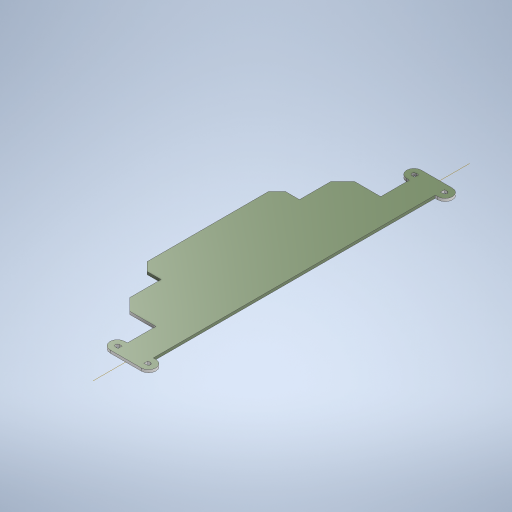
# Autodesk Inventor part: linefollower_chassy_model
Saved by Autodesk Inventor 2024 (Build 280153000, 153)
## iProperties
Created: 2024-02-06
Part Number: linefollower_chassy_model
Material: Generic
Document SubType Name: Modeling
Designer: kamil
Density: 1 g/cm^3
Appearance: Default
Author: kamil
Autodesk Inventor part; units mm, degrees
ref_plane "YZ Plane" through (0, 0, 0) normal (1, 0, 0) x (0, 1, 0)
ref_plane "XZ Plane" through (0, 0, 0) normal (0, 1, 0) x (-1, 0, 0)
ref_plane "XY Plane" through (0, 0, 0) normal (0, 0, 1) x (1, 0, 0)
sketch "Sketch1" plane through (0, 0, 0) normal (0, 1, 0) x (-1, 0, 0)
  line L0 (7.5, 90) -> (-7.5, 90)
  line L1 (-7.5, 90) -> (-7.5, -90)
  line L2 (-7.5, -90) -> (7.5, -90)
  line L3 (7.5, -90) -> (7.5, 90)
  line L4 (-7.5, 90) -> (7.5, -90) construction
  line L5 (-7.5, -90) -> (7.5, 90) construction
  line L6 (7.5, -90) -> (7.5, -81.5)
  line L7 (0, 90) -> (0, -90) construction
  line L8 (-7.5, 0) -> (7.5, 0) construction
  line L9 (7.5, -20.0447) -> (7.5, 20.0447)
  line L10 (7.5, 40) -> (37.5, 40)
  line L11 (42.5, 35) -> (42.5, -35)
  line L12 (37.5, -40) -> (7.5, -40)
  line L13 (7.5, -40) -> (7.5, 40)
  line L14 (-7.5, 1.5) -> (-14.5, 1.5)
  line L15 (-14.5, 1.5) -> (-14.5, -1.5)
  line L16 (-14.5, -1.5) -> (-7.5, -1.5)
  line L17 (-7.5, -1.5) -> (-7.5, 1.5)
  circle A0 centre (-12.5, 0) radius 0.98
  line L18 (37.5, -40) -> (42.5, -35)
  line L19 (37.5, 40) -> (42.5, 35)
  line L20 (7.5, -90) -> (9, -90)
  line L21 (7.5, -81.5) -> (9.01, -81.5)
  arc A1 (9, -90) -> (9.01, -81.5) centre (9.005, -85.75) ccw
  line L22 (7.5, -84.6) -> (9, -84.6)
  line L23 (7.5, -86.9) -> (9, -86.9)
  arc A2 (9, -86.9) -> (9, -84.6) centre (9, -85.75) ccw
  line L24 (-7.5, -90) -> (-9, -90)
  line L25 (-7.5, -81.5) -> (-9.01, -81.5)
  arc A3 (-9.01, -81.5) -> (-9, -90) centre (-9.005, -85.75) ccw
  line L26 (-7.5, -84.6) -> (-9, -84.6)
  line L27 (-7.5, -86.9) -> (-9, -86.9)
  arc A4 (-9, -84.6) -> (-9, -86.9) centre (-9, -85.75) ccw
  arc A5 (9.01, 81.5) -> (9, 90) centre (9.005, 85.75) ccw
  arc A6 (9, 84.6) -> (9, 86.9) centre (9, 85.75) ccw
  arc A7 (-9, 86.9) -> (-9, 84.6) centre (-9, 85.75) ccw
  arc A8 (-9, 90) -> (-9.01, 81.5) centre (-9.005, 85.75) ccw
  line L28 (9, 90) -> (7.5, 90)
  line L29 (9.01, 81.5) -> (7.5, 81.5)
  line L30 (-9, 90) -> (-7.5, 90)
  line L31 (-9.01, 81.5) -> (-7.5, 81.5)
  line L32 (7.5, 65) -> (22.5, 65)
  line L33 (29.5, 58) -> (29.5, -58)
  line L34 (22.5, -65) -> (7.5, -65)
  line L35 (7.5, -65) -> (7.5, 65)
  line L36 (29.5, 58) -> (22.5, 65)
  line L37 (29.5, -58) -> (22.5, -65)
  line L38 (9, 84.6) -> (7.5, 84.6)
  line L39 (9, 86.9) -> (7.5, 86.9)
  line L40 (-9, 86.9) -> (-7.5, 86.9)
  line L41 (-9, 84.6) -> (-7.5, 84.6)
  point P0 (0, 0)
  point P1 (0, 0)
  point P2 (0, 0)
  point P3 (42.5, -40)
  point P4 (42.5, 40)
  point P5 (42.5, 0)
  point P6 (0, 0)
  point P7 (-11, -1.5)
  point P8 (-14.5, 0)
  point P9 (-7.5, 0)
  point P10 (7.5, -40)
  point P11 (8.25, -90)
  point P12 (8.255, -81.5)
  point P13 (-8.25, -90)
  point P14 (-8.255, -81.5)
  point P15 (8.25, 90)
  point P16 (8.255, 81.5)
  point P17 (-8.25, 90)
  point P18 (-8.255, 81.5)
  point P19 (29.5, -65)
  point P20 (29.5, 65)
  point P21 (29.5, 0)
  point P22 (0, 0)
  point P23 (29.5, -40)
  point P24 (7.5, -65)
  point P25 (29.5, 40)
  dimension "d1" = 15
  dimension "d5" = 35
  dimension "d6" = 80
  dimension "d7" = 1.96
  dimension "d8" = 3
  dimension "d9" = 7
  dimension "d10" = 5
  dimension "d11" = 5
  dimension "d12" = 5
  dimension "d13" = 5
  dimension "d14" = 5
  dimension "d17" = 180
  dimension "d18" = 1.5
  dimension "d19" = 1.51
  dimension "d20" = 8.5
  dimension "d21" = 1.5
  dimension "d22" = 3.1
  dimension "d23" = 1.5
  dimension "d24" = 2.3
  dimension "d26" = 130
  dimension "d27" = 22
  dimension "d28" = 7
  dimension "d29" = 7
  dimension "d30" = 7
  dimension "d31" = 7
  constraints: 82 end point, 27 symmetric about line, 16 point on circle, 16 point on line, 14 midpoint, 9 centre point, 9 horizontal, 8 parallel, 7 perpendicular, 4 horizontal alignment, 1 coincident, 1 collinear, 1 vertical, 18 other
  measures "d5" distance of point (42.5, -40) L12.end
  measures "d6" distance of point (42.5, 40) point (42.5, -40)
  measures "d7" diameter of A0
  measures "d8" distance from line of point (-11, -1.5) L14
  measures "d9" distance between parallel lines of L1 L15
  measures "d10" distance of point (-7.5, 0) A0.centre
  measures "d11" distance of L12.start point (42.5, -40)
  measures "d12" distance of L11.end point (42.5, -40)
  measures "d13" distance of L10.end point (42.5, 40)
  measures "d14" distance of L11.start point (42.5, 40)
  measures "d17" distance of L0.end L1.end
  measures "d18" distance of L2.end L20.end
  measures "d19" distance of L21.start L21.end
  measures "d20" distance of point (8.25, -90) point (8.255, -81.5)
  measures "d21" distance of L22.start L22.end
  measures "d22" distance between parallel lines of L22 L21
  measures "d23" distance of L23.start L23.end
  measures "d24" distance between parallel lines of L23 L22
  measures "d26" distance of point (29.5, 65) point (29.5, -65)
  measures "d27" distance of point (29.5, -65) L34.end
  measures "d28" distance of L33.start point (29.5, 65)
  measures "d29" distance of L32.end point (29.5, 65)
  measures "d30" distance of L33.end point (29.5, -65)
  measures "d31" distance of L34.start point (29.5, -65)
extrude "Extrusion1" add sketch "Sketch1" along normal blind 1.57 contours L3 L2 L1 L0 | L28 A5 L29 L3 L38 A6 L39 | L1 L40 A7 L41 L31 A8 L30 | L32 L36 L33 L10 L3 | L10 L33 L12 L3 | L10 L19 L11 L18 L12 L33 | L1 L26 A4 L27 L24 A3 L25 | L33 L37 L34 L3 L12 | L21 A1 L20 L3 L23 A2 L22
equation "\"d12\" = d11"
equation "\"d13\" = d11"
equation "\"d14\" = d13"
equation "\"d29\" = d28"
equation "\"d30\" = d28"
equation "\"d31\" = d30"
body "Solid1"
